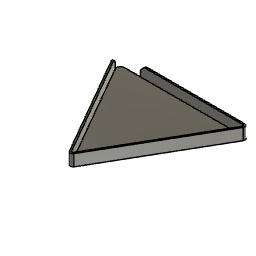
Pill Counter (Autodesk Fusion 360 design; units mm, degrees)
Autodesk Fusion 360 part; units mm, degrees
note: some values were not read from the file. Set by a fixed rule: which sketch regions a step uses.
sketch "Sketch1" plane through (0, 0, 0) normal (0, 0, 1) x (1, 0, 0)
  line L0 (-50, 86.6025) -> (0, 0)
  line L1 (0, 0) -> (50, 86.6025)
  line L2 (50, 86.6025) -> (-50, 86.6025)
  line L3 (52.0785, 87.8025) -> (-52.0785, 87.8025)
  line L4 (-52.0785, 87.8025) -> (0, -2.4)
  line L5 (0, -2.4) -> (52.0785, 87.8025)
  line L6 (-32.0785, 87.8025) -> (-32.0785, 86.6025)
  line L7 (-48.5392, 81.6724) -> (-47.5, 82.2724)
  point P0 (0, 57.735)
  dimension "d1" = 100
  dimension "d2" = 1.2
  dimension "d20" = 20
  dimension "d21" = 5
  constraint horizontal L2
  constraint coincident L0.end L1.start
  constraint coincident L3 L6.start
  constraint coincident L2 L6.end
  constraint perpendicular L2 L6
  constraint coincident L4 L7.start
  constraint coincident L0 L7.end
  constraint perpendicular L0 L7
  measures "d1" distance of L0.start L1.end
  measures "d20" distance of L3.end L6.start
  measures "d21" distance of L0.start L7.end
extrude "Extrude1" add sketch "Sketch1" along normal blind 9
fillet "Fillet3" radius 2 3 edges at (-52.0785, 87.8025, 4.5) (0, -2.4, 4.5) (52.0785, 87.8025, 4.5)
shell "Shell1" thickness 1.2 removed faces 1 at (0.5774, 58.735, 9)
extrude "Extrude3" cut sketch "Sketch1" along normal blind 9 contours L0 L2 L3 L4 L6 L7
fillet "Fillet4" radius 3 1 edges at (-50, 86.6025, 4.5)
chamfer "Chamfer2" distance 3 angle 45 2 edges at (-32.0785, 87.2025, 9) (-48.0196, 81.9724, 9)
named bodies: "Pill Counter"
